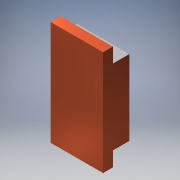
# Autodesk Inventor part: LW-Q38E-Q100-3K6L-1
Saved by Autodesk Inventor 2016 (Build 200138000, 138)
## iProperties
Created: 2016-01-30
Part Number: LW-Q38E-Q100-3K6L-1
Material: Generic
Document SubType Name: Modeling
Designer: jferner
Density: 1 g/cm^3
Appearance: Default
LWQ38EQ1003K6L1_x: 0.800 mm
LWQ38EQ1003K6L1_y: 1.600 mm
Author: jferner
Autodesk Inventor part; units mm, degrees
ref_plane "YZ Plane" through (0, 0, 0) normal (1, 0, 0) x (0, 1, 0)
ref_plane "XZ Plane" through (0, 0, 0) normal (0, 1, 0) x (-1, 0, 0)
ref_plane "XY Plane" through (0, 0, 0) normal (0, 0, 1) x (1, 0, 0)
sketch "Sketch1" plane through (0, 0, 0) normal (0, 1, 0) x (-1, 0, 0)
  line L0 (0, 0) -> (-0.8, 0)
  line L1 (-0.8, 0) -> (-0.8, -1.6)
  line L2 (-0.8, -1.6) -> (0, -1.6)
  line L3 (0, -1.6) -> (0, 0)
  dimension "LWQ38EQ1003K6L1_x" = 0.8
  dimension "LWQ38EQ1003K6L1_y" = 1.6
  constraints: 8 end point, 2 parallel, 1 horizontal, 1 perpendicular
  measures "LWQ38EQ1003K6L1_x" distance of L1.end L2.end
  measures "LWQ38EQ1003K6L1_y" distance of L0.end L1.end
extrude "Extrusion1" add sketch "Sketch1" along normal blind 0.15
sketch "Sketch2" plane through (0, 0.15, 0) normal (0, 1, 0) x (1, 0, 0)
  line L0 (0, 1.6) -> (0, 0) projected
  line L1 (0.8, 0) -> (0.8, 1.6) projected
  line L2 (0, 1.375) -> (0.8, 1.375)
  line L3 (0.8, 1.375) -> (0.8, 0.225)
  line L4 (0.8, 0.225) -> (0, 0.225)
  line L5 (0, 0.225) -> (0, 1.375)
  line L6 (0, 0) -> (0.8, 0) projected
  dimension "d4" = 1.15
  dimension "d5" = 0.225
  constraints: 8 end point, 2 parallel, 2 point on line, 1 horizontal, 1 perpendicular
  measures "d4" distance between parallel lines of L4 L2
  measures "d5" distance between parallel lines of L6 L4
extrude "Extrusion2" add sketch "Sketch2" along normal blind 0.25 contours L2 L1 L4 L0
equation "\"d5\" = -0.5 * d4 + 0.5 * LWQ38EQ1003K6L1_y"
body "Solid1"
